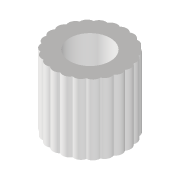
# Autodesk Inventor part: 00_CCTV_Lens_Knob
Saved by Autodesk Inventor 2022.5 (Build 265521000, 521)
## iProperties
Created: 2023-11-21
Part Number: 00_CCTV_Lens_Knob
Material: Generisch
Document SubType Name: Modeling
Designer: diederichbenedict
Density: 1 g/cm^3
Appearance: Vorgabe
Author: diederichbenedict
Autodesk Inventor part; units mm, degrees
ref_plane "YZ Plane" through (0, 0, 0) normal (1, 0, 0) x (0, 1, 0)
ref_plane "XZ Plane" through (0, 0, 0) normal (0, 1, 0) x (-1, 0, 0)
ref_plane "XY Plane" through (0, 0, 0) normal (0, 0, 1) x (1, 0, 0)
sketch "Skizze1" plane through (0, 0, 0) normal (0, 1, 0) x (-1, 0, 0)
  circle A0 centre (0, 0) radius 8.65
  circle A1 centre (0, 0) radius 15
  dimension "d0" = 17.3
  dimension "d1" = 30
  constraints: 2 centre point, 2 coincident
  measures "d0" diameter of A0
  measures "d1" diameter of A1
extrude "Extrusion1" add sketch "Skizze1" along normal blind 30
sketch "Skizze2" plane through (0, 0, 0) normal (1, 0, 0) x (0, 1, 0)
  line L0 (30, -15) -> (30, 15) projected
  line L1 (0, -15) -> (0, 15) projected
  circle A0 centre (3.817, 0) radius 1.4
  point P0 (0, 0)
  dimension "d4" = 2.8
  constraints: 1 centre point
  measures "d4" diameter of A0
extrude "Extrusion2" cut sketch "Skizze2" against normal blind 20
pattern_circular "Runde Anordnung1" count 3 over 360 about axis through (0, 0, 0) along (0, 1, 0) of "Extrusion2"
sketch "Skizze3" plane through (0, 30, 0) normal (0, 1, 0) x (1, 0, 0)
  circle A0 centre (0, 0) radius 15 projected
  circle A1 centre (0, 0) radius 15 projected
  arc A2 (-14.368, 4.3081) -> (-15, 0) centre (-12.5959, 1.8477) ccw
  point P0 (-15, 0)
  point P1 (-14.368, 4.3081)
  constraints: 4 point on circle, 1 centre point
extrude "Extrusion3" add sketch "Skizze3" against normal up to surface (30 mm away) contours A0 A2
pattern_circular "Runde Anordnung2" count 22 over 360 about axis through (0, 0, 0) along (0, 1, 0) of "Extrusion3"
